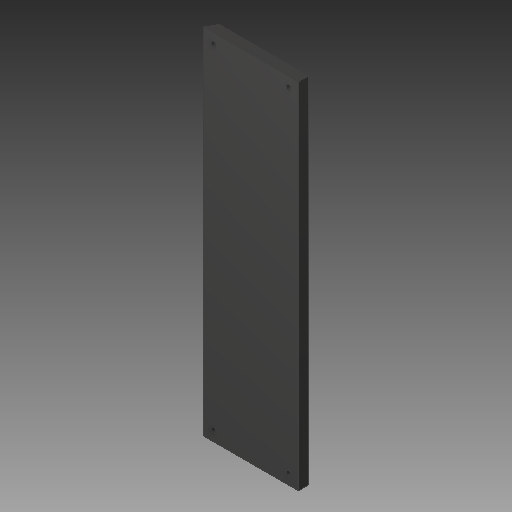
# Autodesk Inventor part: BA09
Saved by Autodesk Inventor 2017 (Build 210142000, 142)
## iProperties
Created: 2018-10-18
Part Number: BA09
Material: ABS Plastic
Document SubType Name: Modeling
Designer: Dell
Density: 1.06 g/cm^3
Appearance: Smooth - Black
Author: Dell
Autodesk Inventor part; units mm, degrees
ref_plane "YZ Plane" through (0, 0, 0) normal (1, 0, 0) x (0, 1, 0)
ref_plane "XZ Plane" through (0, 0, 0) normal (0, 1, 0) x (-1, 0, 0)
ref_plane "XY Plane" through (0, 0, 0) normal (0, 0, 1) x (1, 0, 0)
sketch "Sketch1" plane through (0, 0, 0) normal (0, 0, 1) x (1, 0, 0)
  line L0 (0, 0) -> (95.25, 0)
  line L1 (95.25, 0) -> (95.25, 355.6)
  line L2 (95.25, 355.6) -> (0, 355.6)
  line L3 (0, 355.6) -> (0, 0)
  dimension "d0" = 95.25
  dimension "d1" = 355.6
  constraints: 8 end point, 2 parallel, 1 horizontal, 1 perpendicular
  measures "d0" distance of L2.end L1.end
  measures "d1" distance of L0.end L1.end
extrude "Extrusion1" add sketch "Sketch1" along normal blind 10
sketch "Sketch2" plane through (0, 355.6, 0) normal (0, 1, 0) x (1, 0, 0)
  line L0 (0, -10) -> (95.25, -10) projected
  line L1 (0, -10) -> (5.7735, 0)
  line L2 (0, 0) -> (95.25, 0) projected
  line L3 (0, 0) -> (0, -10)
  line L4 (5.7735, 0) -> (0, 0)
  dimension "d4" = 30
  constraints: 6 end point, 1 perpendicular, 1 point on line, 1 vertical
  measures "d4" angle of L3 L1
extrude "Extrusion2" cut sketch "Sketch2" against normal blind 355.6
sketch "Sketch3" plane through (0, 0, 10) normal (0, 0, 1) x (1, 0, 0)
  line L0 (0, 0) -> (95.25, 0) construction
  line L1 (95.25, 0) -> (95.25, 355.6) construction
  line L2 (95.25, 355.6) -> (0, 355.6) construction
  line L3 (0, 355.6) -> (0, 0) construction
  line L4 (10, 10) -> (85.25, 10) construction
  line L5 (85.25, 10) -> (85.25, 345.6) construction
  line L6 (85.25, 345.6) -> (10, 345.6) construction
  line L7 (10, 345.6) -> (10, 10) construction
  circle A0 centre (10, 345.6) radius 2.5
  circle A1 centre (85.25, 345.6) radius 2.5
  circle A2 centre (85.25, 10) radius 2.5
  circle A3 centre (10, 10) radius 2.5
  dimension "d7" = 10
  dimension "d8" = 5
  dimension "d9" = 5
  dimension "d10" = 5
  dimension "d11" = 5
  constraints: 8 end point, 4 centre point, 4 coincident, 3 other
  measures "d7" distance between parallel lines of L3 L7
  measures "d8" diameter of A0
  measures "d9" diameter of A1
  measures "d10" diameter of A2
  measures "d11" diameter of A3
extrude "Extrusion3" cut sketch "Sketch3" against normal through all
body "Solid1"
